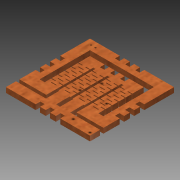
# Autodesk Inventor part: mech
Saved by Autodesk Inventor 2014 SP1 (Build 180222100, 222)
## iProperties
Created: 2015-02-17
Part Number: mech
Material: Wood (Cherry)
Document SubType Name: Modeling
Designer: Erin
Density: 0.63 g/cm^3
Appearance: Cherry - Natural Low Gloss
Author: Erin
Autodesk Inventor part; units mm, degrees
(part 1 of 2)
ref_plane "YZ Plane" through (0, 0, 0) normal (1, 0, 0) x (0, 1, 0)
ref_plane "XZ Plane" through (0, 0, 0) normal (0, 1, 0) x (-1, 0, 0)
ref_plane "XY Plane" through (0, 0, 0) normal (0, 0, 1) x (1, 0, 0)
sketch "slots" plane through (0, 0, 0) normal (0, 0, 1) x (1, 0, 0)
  line L0 (61.2067, 31.1821) -> (64.2567, 31.1821)
  line L1 (64.2567, 31.1821) -> (64.2567, 28.1071)
  line L2 (64.2567, 28.1071) -> (61.2067, 28.1071)
  line L3 (61.2067, 28.1071) -> (61.2067, 31.1821)
  line L4 (68.9317, 33.8834) -> (68.9317, 26.9198) construction
  line L5 (67.4067, 31.1821) -> (70.4567, 31.1821)
  line L6 (70.4567, 31.1821) -> (70.4567, 28.1071)
  line L7 (70.4567, 28.1071) -> (67.4067, 28.1071)
  line L8 (67.4067, 28.1071) -> (67.4067, 31.1821)
  line L9 (73.6067, 31.1821) -> (76.6567, 31.1821)
  line L10 (76.6567, 31.1821) -> (76.6567, 28.1071)
  line L11 (76.6567, 28.1071) -> (73.6067, 28.1071)
  line L12 (73.6067, 28.1071) -> (73.6067, 31.1821)
  line L13 (68.9317, 28.1071) -> (68.9317, 27.1937) construction
  point P0 (68.8645, 30.3856)
  dimension "d2" = 3.05
  dimension "d3" = 3.075
  dimension "d99" = 3.15
  dimension "d100" = 3.15
  measures "d2" distance of L1.end L2.end
  measures "d3" distance of L0.end L1.end
  measures "d99" distance between parallel lines of L8 L1
  measures "d100" distance between parallel lines of L12 L6
sketch "flexure" plane through (0, 0, 0) normal (0, 0, 1) x (1, 0, 0)
  line L0 (48.9032, 41.5133) -> (55.9032, 41.5133)
  line L1 (55.9032, 41.5133) -> (55.9032, 19.5133)
  line L2 (55.9032, 19.5133) -> (48.9032, 19.5133)
  line L3 (48.9032, 19.5133) -> (48.9032, 41.5133)
  line L4 (48.9032, 31.7633) -> (51.4486, 31.7633)
  line L5 (51.4486, 31.7633) -> (51.4486, 31.2633)
  line L6 (51.4486, 31.2633) -> (48.9032, 31.2633)
  line L7 (48.9032, 31.2633) -> (48.9032, 31.7633)
  line L8 (53.3577, 31.2633) -> (53.3577, 31.7633)
  line L9 (55.9032, 31.2633) -> (53.3577, 31.2633)
  line L10 (53.3577, 31.7633) -> (55.9032, 31.7633)
  line L11 (55.9032, 31.7633) -> (55.9032, 31.2633)
  line L12 (50.8123, 29.7633) -> (53.9941, 29.7633)
  line L13 (53.9941, 29.7633) -> (53.9941, 29.2633)
  line L14 (53.9941, 29.2633) -> (50.8123, 29.2633)
  line L15 (50.8123, 29.2633) -> (50.8123, 29.7633)
  line L16 (48.9032, 30.5133) -> (55.9032, 30.5133) construction
  line L17 (55.9032, 30.5133) -> (48.9032, 30.5133) construction
  line L18 (53.3577, 27.7633) -> (55.9032, 27.7633)
  line L19 (55.9032, 27.7633) -> (55.9032, 27.2633)
  line L20 (55.9032, 27.2633) -> (53.3577, 27.2633)
  line L21 (53.3577, 27.2633) -> (53.3577, 27.7633)
  line L22 (50.8123, 25.7633) -> (53.9941, 25.7633)
  line L23 (53.9941, 25.7633) -> (53.9941, 25.2633)
  line L24 (53.9941, 25.2633) -> (50.8123, 25.2633)
  line L25 (50.8123, 25.2633) -> (50.8123, 25.7633)
  line L26 (48.9032, 27.7633) -> (51.4486, 27.7633)
  line L27 (51.4486, 27.7633) -> (51.4486, 27.2633)
  line L28 (51.4486, 27.2633) -> (48.9032, 27.2633)
  line L29 (48.9032, 27.2633) -> (48.9032, 27.7633)
  line L30 (48.9032, 26.5133) -> (55.9032, 26.5133) construction
  line L31 (55.9032, 26.5133) -> (48.9032, 26.5133) construction
  line L32 (53.3577, 23.7633) -> (55.9032, 23.7633)
  line L33 (55.9032, 23.7633) -> (55.9032, 23.2633)
  line L34 (55.9032, 23.2633) -> (53.3577, 23.2633)
  line L35 (53.3577, 23.2633) -> (53.3577, 23.7633)
  line L36 (50.8123, 21.7633) -> (53.9941, 21.7633)
  line L37 (53.9941, 21.7633) -> (53.9941, 21.2633)
  line L38 (53.9941, 21.2633) -> (50.8123, 21.2633)
  line L39 (50.8123, 21.2633) -> (50.8123, 21.7633)
  line L40 (48.9032, 23.7633) -> (51.4486, 23.7633)
  line L41 (51.4486, 23.7633) -> (51.4486, 23.2633)
  line L42 (51.4486, 23.2633) -> (48.9032, 23.2633)
  line L43 (48.9032, 23.2633) -> (48.9032, 23.7633)
  line L44 (48.9032, 22.5133) -> (55.9032, 22.5133) construction
  line L45 (55.9032, 22.5133) -> (48.9032, 22.5133) construction
  line L46 (53.3577, 35.7633) -> (55.9032, 35.7633)
  line L47 (55.9032, 35.7633) -> (55.9032, 35.2633)
  line L48 (55.9032, 35.2633) -> (53.3577, 35.2633)
  line L49 (53.3577, 35.2633) -> (53.3577, 35.7633)
  line L50 (50.8123, 33.7633) -> (53.9941, 33.7633)
  line L51 (53.9941, 33.7633) -> (53.9941, 33.2633)
  line L52 (53.9941, 33.2633) -> (50.8123, 33.2633)
  line L53 (50.8123, 33.2633) -> (50.8123, 33.7633)
  line L54 (48.9032, 35.7633) -> (51.4486, 35.7633)
  line L55 (51.4486, 35.7633) -> (51.4486, 35.2633)
  line L56 (51.4486, 35.2633) -> (48.9032, 35.2633)
  line L57 (48.9032, 35.2633) -> (48.9032, 35.7633)
  line L58 (48.9032, 34.5133) -> (55.9032, 34.5133) construction
  line L59 (55.9032, 34.5133) -> (48.9032, 34.5133) construction
  line L60 (53.3577, 31.7633) -> (55.9032, 31.7633)
  line L61 (55.9032, 31.7633) -> (55.9032, 31.2633)
  line L62 (55.9032, 31.2633) -> (53.3577, 31.2633)
  line L63 (53.3577, 31.2633) -> (53.3577, 31.7633)
  line L64 (50.8123, 29.7633) -> (53.9941, 29.7633)
  line L65 (53.9941, 29.7633) -> (53.9941, 29.2633)
  line L66 (53.9941, 29.2633) -> (50.8123, 29.2633)
  line L67 (50.8123, 29.2633) -> (50.8123, 29.7633)
  line L68 (48.9032, 31.7633) -> (51.4486, 31.7633)
  line L69 (51.4486, 31.7633) -> (51.4486, 31.2633)
  line L70 (51.4486, 31.2633) -> (48.9032, 31.2633)
  line L71 (48.9032, 31.2633) -> (48.9032, 31.7633)
  line L72 (48.9032, 30.5133) -> (55.9032, 30.5133) construction
  line L73 (55.9032, 30.5133) -> (48.9032, 30.5133) construction
  line L74 (53.3577, 27.7633) -> (55.9032, 27.7633)
  line L75 (55.9032, 27.7633) -> (55.9032, 27.2633)
  line L76 (55.9032, 27.2633) -> (53.3577, 27.2633)
  line L77 (53.3577, 27.2633) -> (53.3577, 27.7633)
  line L78 (50.8123, 25.7633) -> (53.9941, 25.7633)
  line L79 (53.9941, 25.7633) -> (53.9941, 25.2633)
  line L80 (53.9941, 25.2633) -> (50.8123, 25.2633)
  line L81 (50.8123, 25.2633) -> (50.8123, 25.7633)
  line L82 (48.9032, 27.7633) -> (51.4486, 27.7633)
  line L83 (51.4486, 27.7633) -> (51.4486, 27.2633)
  line L84 (51.4486, 27.2633) -> (48.9032, 27.2633)
  line L85 (48.9032, 27.2633) -> (48.9032, 27.7633)
  line L86 (48.9032, 26.5133) -> (55.9032, 26.5133) construction
  line L87 (55.9032, 26.5133) -> (48.9032, 26.5133) construction
  line L88 (53.3577, 39.7633) -> (55.9032, 39.7633)
  line L89 (55.9032, 39.7633) -> (55.9032, 39.2633)
  line L90 (55.9032, 39.2633) -> (53.3577, 39.2633)
  line L91 (53.3577, 39.2633) -> (53.3577, 39.7633)
  line L92 (50.8123, 37.7633) -> (53.9941, 37.7633)
  line L93 (53.9941, 37.7633) -> (53.9941, 37.2633)
  line L94 (53.9941, 37.2633) -> (50.8123, 37.2633)
  line L95 (50.8123, 37.2633) -> (50.8123, 37.7633)
  line L96 (48.9032, 39.7633) -> (51.4486, 39.7633)
  line L97 (51.4486, 39.7633) -> (51.4486, 39.2633)
  line L98 (51.4486, 39.2633) -> (48.9032, 39.2633)
  line L99 (48.9032, 39.2633) -> (48.9032, 39.7633)
  line L100 (48.9032, 38.5133) -> (55.9032, 38.5133) construction
  line L101 (55.9032, 38.5133) -> (48.9032, 38.5133) construction
  line L102 (53.3577, 35.7633) -> (55.9032, 35.7633)
  line L103 (55.9032, 35.7633) -> (55.9032, 35.2633)
  line L104 (55.9032, 35.2633) -> (53.3577, 35.2633)
  line L105 (53.3577, 35.2633) -> (53.3577, 35.7633)
  line L106 (50.8123, 33.7633) -> (53.9941, 33.7633)
  line L107 (53.9941, 33.7633) -> (53.9941, 33.2633)
  line L108 (53.9941, 33.2633) -> (50.8123, 33.2633)
  line L109 (50.8123, 33.2633) -> (50.8123, 33.7633)
  line L110 (48.9032, 35.7633) -> (51.4486, 35.7633)
  line L111 (51.4486, 35.7633) -> (51.4486, 35.2633)
  line L112 (51.4486, 35.2633) -> (48.9032, 35.2633)
  line L113 (48.9032, 35.2633) -> (48.9032, 35.7633)
  line L114 (48.9032, 34.5133) -> (55.9032, 34.5133) construction
  line L115 (55.9032, 34.5133) -> (48.9032, 34.5133) construction
  line L116 (53.3577, 31.7633) -> (55.9032, 31.7633)
  line L117 (55.9032, 31.7633) -> (55.9032, 31.2633)
  line L118 (55.9032, 31.2633) -> (53.3577, 31.2633)
  line L119 (53.3577, 31.2633) -> (53.3577, 31.7633)
  line L120 (50.8123, 29.7633) -> (53.9941, 29.7633)
  line L121 (53.9941, 29.7633) -> (53.9941, 29.2633)
  line L122 (53.9941, 29.2633) -> (50.8123, 29.2633)
  line L123 (50.8123, 29.2633) -> (50.8123, 29.7633)
  line L124 (48.9032, 31.7633) -> (51.4486, 31.7633)
  line L125 (51.4486, 31.7633) -> (51.4486, 31.2633)
  line L126 (51.4486, 31.2633) -> (48.9032, 31.2633)
  line L127 (48.9032, 31.2633) -> (48.9032, 31.7633)
  line L128 (48.9032, 30.5133) -> (55.9032, 30.5133) construction
  line L129 (55.9032, 30.5133) -> (48.9032, 30.5133) construction
  line L130 (53.3577, 19.7633) -> (55.9032, 19.7633)
  line L131 (55.9032, 19.7633) -> (55.9032, 19.2633)
  line L132 (55.9032, 19.2633) -> (53.3577, 19.2633)
  line L133 (53.3577, 19.2633) -> (53.3577, 19.7633)
  line L134 (50.8123, 17.7633) -> (53.9941, 17.7633)
  line L135 (53.9941, 17.7633) -> (53.9941, 17.2633)
  line L136 (53.9941, 17.2633) -> (50.8123, 17.2633)
  line L137 (50.8123, 17.2633) -> (50.8123, 17.7633)
  line L138 (48.9032, 19.7633) -> (51.4486, 19.7633)
  line L139 (51.4486, 19.7633) -> (51.4486, 19.2633)
  line L140 (51.4486, 19.2633) -> (48.9032, 19.2633)
  line L141 (48.9032, 19.2633) -> (48.9032, 19.7633)
  line L142 (48.9032, 18.5133) -> (55.9032, 18.5133) construction
  line L143 (55.9032, 18.5133) -> (48.9032, 18.5133) construction
  line L144 (53.3577, 23.7633) -> (55.9032, 23.7633)
  line L145 (55.9032, 23.7633) -> (55.9032, 23.2633)
  line L146 (55.9032, 23.2633) -> (53.3577, 23.2633)
  line L147 (53.3577, 23.2633) -> (53.3577, 23.7633)
  line L148 (50.8123, 21.7633) -> (53.9941, 21.7633)
  line L149 (53.9941, 21.7633) -> (53.9941, 21.2633)
  line L150 (53.9941, 21.2633) -> (50.8123, 21.2633)
  line L151 (50.8123, 21.2633) -> (50.8123, 21.7633)
  line L152 (48.9032, 23.7633) -> (51.4486, 23.7633)
  line L153 (51.4486, 23.7633) -> (51.4486, 23.2633)
  line L154 (51.4486, 23.2633) -> (48.9032, 23.2633)
  line L155 (48.9032, 23.2633) -> (48.9032, 23.7633)
  line L156 (48.9032, 22.5133) -> (55.9032, 22.5133) construction
  line L157 (55.9032, 22.5133) -> (48.9032, 22.5133) construction
  line L158 (53.3577, 27.7633) -> (55.9032, 27.7633)
  line L159 (55.9032, 27.7633) -> (55.9032, 27.2633)
  line L160 (55.9032, 27.2633) -> (53.3577, 27.2633)
  line L161 (53.3577, 27.2633) -> (53.3577, 27.7633)
  line L162 (50.8123, 25.7633) -> (53.9941, 25.7633)
  line L163 (53.9941, 25.7633) -> (53.9941, 25.2633)
  line L164 (53.9941, 25.2633) -> (50.8123, 25.2633)
  line L165 (50.8123, 25.2633) -> (50.8123, 25.7633)
  line L166 (48.9032, 27.7633) -> (51.4486, 27.7633)
  line L167 (51.4486, 27.7633) -> (51.4486, 27.2633)
  line L168 (51.4486, 27.2633) -> (48.9032, 27.2633)
  line L169 (48.9032, 27.2633) -> (48.9032, 27.7633)
  line L170 (48.9032, 26.5133) -> (55.9032, 26.5133) construction
  line L171 (55.9032, 26.5133) -> (48.9032, 26.5133) construction
  line L172 (53.3577, 43.7633) -> (55.9032, 43.7633)
  line L173 (55.9032, 43.7633) -> (55.9032, 43.2633)
  line L174 (55.9032, 43.2633) -> (53.3577, 43.2633)
  line L175 (53.3577, 43.2633) -> (53.3577, 43.7633)
  line L176 (50.8123, 41.7633) -> (53.9941, 41.7633)
  line L177 (53.9941, 41.7633) -> (53.9941, 41.2633)
  line L178 (53.9941, 41.2633) -> (50.8123, 41.2633)
  line L179 (50.8123, 41.2633) -> (50.8123, 41.7633)
  line L180 (48.9032, 43.7633) -> (51.4486, 43.7633)
  line L181 (51.4486, 43.7633) -> (51.4486, 43.2633)
  line L182 (51.4486, 43.2633) -> (48.9032, 43.2633)
  line L183 (48.9032, 43.2633) -> (48.9032, 43.7633)
  line L184 (48.9032, 42.5133) -> (55.9032, 42.5133) construction
  line L185 (55.9032, 42.5133) -> (48.9032, 42.5133) construction
  line L186 (53.3577, 39.7633) -> (55.9032, 39.7633)
  line L187 (55.9032, 39.7633) -> (55.9032, 39.2633)
  line L188 (55.9032, 39.2633) -> (53.3577, 39.2633)
  line L189 (53.3577, 39.2633) -> (53.3577, 39.7633)
  line L190 (50.8123, 37.7633) -> (53.9941, 37.7633)
  line L191 (53.9941, 37.7633) -> (53.9941, 37.2633)
  line L192 (53.9941, 37.2633) -> (50.8123, 37.2633)
  line L193 (50.8123, 37.2633) -> (50.8123, 37.7633)
  line L194 (48.9032, 39.7633) -> (51.4486, 39.7633)
  line L195 (51.4486, 39.7633) -> (51.4486, 39.2633)
  line L196 (51.4486, 39.2633) -> (48.9032, 39.2633)
  line L197 (48.9032, 39.2633) -> (48.9032, 39.7633)
  line L198 (48.9032, 38.5133) -> (55.9032, 38.5133) construction
  line L199 (55.9032, 38.5133) -> (48.9032, 38.5133) construction
  line L200 (53.3577, 35.7633) -> (55.9032, 35.7633)
  line L201 (55.9032, 35.7633) -> (55.9032, 35.2633)
  line L202 (55.9032, 35.2633) -> (53.3577, 35.2633)
  line L203 (53.3577, 35.2633) -> (53.3577, 35.7633)
  line L204 (50.8123, 33.7633) -> (53.9941, 33.7633)
  line L205 (53.9941, 33.7633) -> (53.9941, 33.2633)
  line L206 (53.9941, 33.2633) -> (50.8123, 33.2633)
  line L207 (50.8123, 33.2633) -> (50.8123, 33.7633)
  line L208 (48.9032, 35.7633) -> (51.4486, 35.7633)
  line L209 (51.4486, 35.7633) -> (51.4486, 35.2633)
  line L210 (51.4486, 35.2633) -> (48.9032, 35.2633)
  line L211 (48.9032, 35.2633) -> (48.9032, 35.7633)
  line L212 (48.9032, 34.5133) -> (55.9032, 34.5133) construction
  line L213 (55.9032, 34.5133) -> (48.9032, 34.5133) construction
  line L214 (53.3577, 31.7633) -> (55.9032, 31.7633)
  line L215 (55.9032, 31.7633) -> (55.9032, 31.2633)
  line L216 (55.9032, 31.2633) -> (53.3577, 31.2633)
  line L217 (53.3577, 31.2633) -> (53.3577, 31.7633)
  line L218 (50.8123, 29.7633) -> (53.9941, 29.7633)
  line L219 (53.9941, 29.7633) -> (53.9941, 29.2633)
  line L220 (53.9941, 29.2633) -> (50.8123, 29.2633)
  line L221 (50.8123, 29.2633) -> (50.8123, 29.7633)
  line L222 (48.9032, 31.7633) -> (51.4486, 31.7633)
  line L223 (51.4486, 31.7633) -> (51.4486, 31.2633)
  line L224 (51.4486, 31.2633) -> (48.9032, 31.2633)
  line L225 (48.9032, 31.2633) -> (48.9032, 31.7633)
  line L226 (48.9032, 30.5133) -> (55.9032, 30.5133) construction
  line L227 (55.9032, 30.5133) -> (48.9032, 30.5133) construction
  point P0 (52.8239, 25.8216)
  dimension "d22" = 7
  dimension "d24" = 2.5455
  dimension "d27" = 4.4546
  dimension "d32" = 1.9091
  dimension "d33" = 3.1818
  dimension "d41" = 0.5
  dimension "d42" = 0.5
  dimension "d43" = 1.5
  dimension "d93" = 22
  dimension "d106" = 4
  dimension "d109" = 4
  dimension "d116" = 11.75
  measures "d22" distance of L1.end L2.end
  measures "d24" distance of L4.start L4.end
  measures "d27" distance of L6.end L9.end
  measures "d32" distance between parallel lines of L15 L3
  measures "d33" distance of L12.start L12.end
  measures "d41" distance of L4.end L5.end
  measures "d42" distance of L12.end L13.end
  measures "d43" distance between parallel lines of L12 L6
  measures "d93" distance of L0.end L1.end
  measures "d106" distance of L10.start L18.start
  measures "d109" distance of L10.start L46.start
  measures "d116" distance between parallel lines of L12 L0
sketch "Sketch1" plane through (0, 0, 0) normal (0, 0, 1) x (1, 0, 0)
  line L0 (-25, 25) -> (25, 25) construction
  line L1 (25, 25) -> (25, -25) construction
  line L2 (25, -25) -> (-25, -25) construction
  line L3 (-25, -25) -> (-25, 25) construction
  line L4 (-25, -25) -> (25, -25)
  line L5 (25, -25) -> (25, -19)
  line L6 (25, -19) -> (-25, -19)
  line L7 (-25, -19) -> (-25, -25)
  line L8 (0, 33.5916) -> (0, -39.9789) construction
  line L9 (-35.9054, 0) -> (42.6007, 0) construction
  line L10 (-25, 25) -> (25, 25)
  line L11 (25, 25) -> (25, 19)
  line L12 (25, 19) -> (-25, 19)
  line L13 (-25, 19) -> (-25, 25)
  line L14 (-25, 19) -> (-19, 19)
  line L15 (-19, 19) -> (-19, -17)
  line L16 (-19, -17) -> (-25, -17)
  line L17 (-25, -17) -> (-25, 19)
  line L18 (-19, -17) -> (-9, -17)
  line L19 (-9, -17) -> (-9, -11)
  line L20 (-9, -11) -> (-19, -11)
  line L21 (-19, -11) -> (-19, -17)
  line L22 (25, 19) -> (19, 19)
  line L23 (19, 19) -> (19, -17)
  line L24 (19, -17) -> (25, -17)
  line L25 (25, -17) -> (25, 19)
  line L26 (19, -17) -> (9, -17)
  line L27 (9, -17) -> (9, -11)
  line L28 (9, -11) -> (19, -11)
  line L29 (19, -11) -> (19, -17)
  line L30 (-16, 16) -> (16, 16)
  line L31 (16, 16) -> (16, 11)
  line L32 (16, 11) -> (-16, 11)
  line L33 (-16, 11) -> (-16, 16)
  line L34 (-7.2, -11) -> (-1.2, -11)
  line L35 (-1.2, -11) -> (-1.2, -19)
  line L36 (-1.2, -19) -> (-7.2, -19)
  line L37 (-7.2, -19) -> (-7.2, -11)
  line L38 (1.2, -11) -> (7.2, -11)
  line L39 (7.2, -11) -> (7.2, -19)
  line L40 (7.2, -19) -> (1.2, -19)
  line L41 (1.2, -19) -> (1.2, -11)
  line L42 (-68.1542, 16.5688) -> (-29.44, 16.5688) construction
  line L43 (-29.44, 16.5688) -> (-29.44, -5.0786) construction
  line L44 (-29.44, -5.0786) -> (-68.1542, -5.0786) construction
  line L45 (-68.1542, -5.0786) -> (-68.1542, 16.5688) construction
  circle A0 centre (-21.2866, 22) radius 0.5
  circle A1 centre (-18.6754, 22) radius 0.5
  line L46 (-7.725, 25) -> (-4.675, 25)
  line L47 (-4.675, 25) -> (-4.675, 21.925)
  line L48 (-4.675, 21.925) -> (-7.725, 21.925)
  line L49 (-7.725, 21.925) -> (-7.725, 25)
  line L50 (0, 27.7013) -> (0, 20.7377) construction
  line L51 (-1.525, 25) -> (1.525, 25)
  line L52 (1.525, 25) -> (1.525, 21.925)
  line L53 (1.525, 21.925) -> (-1.525, 21.925)
  line L54 (-1.525, 21.925) -> (-1.525, 25)
  line L55 (4.675, 25) -> (7.725, 25)
  line L56 (7.725, 25) -> (7.725, 21.925)
  line L57 (7.725, 21.925) -> (4.675, 21.925)
  line L58 (4.675, 21.925) -> (4.675, 25)
  line L59 (0, 21.925) -> (0, 21.0116) construction
  line L60 (-7.725, -21.925) -> (-4.675, -21.925)
  line L61 (-4.675, -21.925) -> (-4.675, -25)
  line L62 (-4.675, -25) -> (-7.725, -25)
  line L63 (-7.725, -25) -> (-7.725, -21.925)
  line L64 (0, -19.2237) -> (0, -26.1873) construction
  line L65 (-1.525, -21.925) -> (1.525, -21.925)
  line L66 (1.525, -21.925) -> (1.525, -25)
  line L67 (1.525, -25) -> (-1.525, -25)
  line L68 (-1.525, -25) -> (-1.525, -21.925)
  line L69 (4.675, -21.925) -> (7.725, -21.925)
  line L70 (7.725, -21.925) -> (7.725, -25)
  line L71 (7.725, -25) -> (4.675, -25)
  line L72 (4.675, -25) -> (4.675, -21.925)
  line L73 (0, -25) -> (0, -25.9134) construction
  line L74 (-25, -7.725) -> (-25, -4.675)
  line L75 (-25, -4.675) -> (-21.925, -4.675)
  line L76 (-21.925, -4.675) -> (-21.925, -7.725)
  line L77 (-21.925, -7.725) -> (-25, -7.725)
  line L78 (-27.7013, 0) -> (-20.7377, 0) construction
  line L79 (-25, -1.525) -> (-25, 1.525)
  line L80 (-25, 1.525) -> (-21.925, 1.525)
  line L81 (-21.925, 1.525) -> (-21.925, -1.525)
  line L82 (-21.925, -1.525) -> (-25, -1.525)
  line L83 (-25, 4.675) -> (-25, 7.725)
  line L84 (-25, 7.725) -> (-21.925, 7.725)
  line L85 (-21.925, 7.725) -> (-21.925, 4.675)
  line L86 (-21.925, 4.675) -> (-25, 4.675)
  line L87 (-21.925, 0) -> (-21.0116, 0) construction
  line L88 (21.925, -7.725) -> (21.925, -4.675)
  line L89 (21.925, -4.675) -> (25, -4.675)
  line L90 (25, -4.675) -> (25, -7.725)
  line L91 (25, -7.725) -> (21.925, -7.725)
  line L92 (19.2237, 0) -> (26.1873, 0) construction
  line L93 (21.925, -1.525) -> (21.925, 1.525)
  line L94 (21.925, 1.525) -> (25, 1.525)
  line L95 (25, 1.525) -> (25, -1.525)
  line L96 (25, -1.525) -> (21.925, -1.525)
  line L97 (21.925, 4.675) -> (21.925, 7.725)
  line L98 (21.925, 7.725) -> (25, 7.725)
  line L99 (25, 7.725) -> (25, 4.675)
  line L100 (25, 4.675) -> (21.925, 4.675)
  line L101 (25, 0) -> (25.9134, 0) construction
  line L102 (-16, 11) -> (-9, 11)
  line L103 (-9, 11) -> (-9, -11)
  line L104 (-9, -11) -> (-16, -11)
  line L105 (-16, -11) -> (-16, 11)
  line L106 (-16, 1.25) -> (-13.4545, 1.25)
  line L107 (-13.4545, 1.25) -> (-13.4545, 0.75)
  line L108 (-13.4545, 0.75) -> (-16, 0.75)
  line L109 (-16, 0.75) -> (-16, 1.25)
  line L110 (-11.5455, 0.75) -> (-11.5455, 1.25)
  line L111 (-9, 0.75) -> (-11.5455, 0.75)
  line L112 (-11.5455, 1.25) -> (-9, 1.25)
  line L113 (-9, 1.25) -> (-9, 0.75)
  line L114 (-14.0909, -0.75) -> (-10.9091, -0.75)
  line L115 (-10.9091, -0.75) -> (-10.9091, -1.25)
  line L116 (-10.9091, -1.25) -> (-14.0909, -1.25)
  line L117 (-14.0909, -1.25) -> (-14.0909, -0.75)
  line L118 (-16, 0) -> (-9, 0) construction
  line L119 (-9, 0) -> (-16, 0) construction
  line L120 (-11.5455, -2.75) -> (-9, -2.75)
  line L121 (-9, -2.75) -> (-9, -3.25)
  line L122 (-9, -3.25) -> (-11.5455, -3.25)
  line L123 (-11.5455, -3.25) -> (-11.5455, -2.75)
  line L124 (-14.0909, -4.75) -> (-10.9091, -4.75)
  line L125 (-10.9091, -4.75) -> (-10.9091, -5.25)
  line L126 (-10.9091, -5.25) -> (-14.0909, -5.25)
  line L127 (-14.0909, -5.25) -> (-14.0909, -4.75)
  line L128 (-16, -2.75) -> (-13.4545, -2.75)
  line L129 (-13.4545, -2.75) -> (-13.4545, -3.25)
  line L130 (-13.4545, -3.25) -> (-16, -3.25)
  line L131 (-16, -3.25) -> (-16, -2.75)
  line L132 (-16, -4) -> (-9, -4) construction
  line L133 (-9, -4) -> (-16, -4) construction
  line L134 (-11.5455, -6.75) -> (-9, -6.75)
  line L135 (-9, -6.75) -> (-9, -7.25)
  line L136 (-9, -7.25) -> (-11.5455, -7.25)
  line L137 (-11.5455, -7.25) -> (-11.5455, -6.75)
  line L138 (-14.0909, -8.75) -> (-10.9091, -8.75)
  line L139 (-10.9091, -8.75) -> (-10.9091, -9.25)
  line L140 (-10.9091, -9.25) -> (-14.0909, -9.25)
  line L141 (-14.0909, -9.25) -> (-14.0909, -8.75)
  line L142 (-16, -6.75) -> (-13.4545, -6.75)
  line L143 (-13.4545, -6.75) -> (-13.4545, -7.25)
  line L144 (-13.4545, -7.25) -> (-16, -7.25)
  line L145 (-16, -7.25) -> (-16, -6.75)
  line L146 (-16, -8) -> (-9, -8) construction
  line L147 (-9, -8) -> (-16, -8) construction
  line L148 (-11.5455, 5.25) -> (-9, 5.25)
  line L149 (-9, 5.25) -> (-9, 4.75)
  line L150 (-9, 4.75) -> (-11.5455, 4.75)
  line L151 (-11.5455, 4.75) -> (-11.5455, 5.25)
  line L152 (-14.0909, 3.25) -> (-10.9091, 3.25)
  line L153 (-10.9091, 3.25) -> (-10.9091, 2.75)
  line L154 (-10.9091, 2.75) -> (-14.0909, 2.75)
  line L155 (-14.0909, 2.75) -> (-14.0909, 3.25)
  line L156 (-16, 5.25) -> (-13.4545, 5.25)
  line L157 (-13.4545, 5.25) -> (-13.4545, 4.75)
  line L158 (-13.4545, 4.75) -> (-16, 4.75)
  line L159 (-16, 4.75) -> (-16, 5.25)
  line L160 (-16, 4) -> (-9, 4) construction
  line L161 (-9, 4) -> (-16, 4) construction
  line L162 (-11.5455, 1.25) -> (-9, 1.25)
  line L163 (-9, 1.25) -> (-9, 0.75)
  line L164 (-9, 0.75) -> (-11.5455, 0.75)
  line L165 (-11.5455, 0.75) -> (-11.5455, 1.25)
  line L166 (-14.0909, -0.75) -> (-10.9091, -0.75)
  line L167 (-10.9091, -0.75) -> (-10.9091, -1.25)
  line L168 (-10.9091, -1.25) -> (-14.0909, -1.25)
  line L169 (-14.0909, -1.25) -> (-14.0909, -0.75)
  line L170 (-16, 1.25) -> (-13.4545, 1.25)
  line L171 (-13.4545, 1.25) -> (-13.4545, 0.75)
  line L172 (-13.4545, 0.75) -> (-16, 0.75)
  line L173 (-16, 0.75) -> (-16, 1.25)
  line L174 (-16, 0) -> (-9, 0) construction
  line L175 (-9, 0) -> (-16, 0) construction
  line L176 (-11.5455, -2.75) -> (-9, -2.75)
  line L177 (-9, -2.75) -> (-9, -3.25)
  line L178 (-9, -3.25) -> (-11.5455, -3.25)
  line L179 (-11.5455, -3.25) -> (-11.5455, -2.75)
  line L180 (-14.0909, -4.75) -> (-10.9091, -4.75)
  line L181 (-10.9091, -4.75) -> (-10.9091, -5.25)
  line L182 (-10.9091, -5.25) -> (-14.0909, -5.25)
  line L183 (-14.0909, -5.25) -> (-14.0909, -4.75)
  line L184 (-16, -2.75) -> (-13.4545, -2.75)
  line L185 (-13.4545, -2.75) -> (-13.4545, -3.25)
  line L186 (-13.4545, -3.25) -> (-16, -3.25)
  line L187 (-16, -3.25) -> (-16, -2.75)
  line L188 (-16, -4) -> (-9, -4) construction
  line L189 (-9, -4) -> (-16, -4) construction
  line L190 (-11.5455, 9.25) -> (-9, 9.25)
  line L191 (-9, 9.25) -> (-9, 8.75)
  line L192 (-9, 8.75) -> (-11.5455, 8.75)
  line L193 (-11.5455, 8.75) -> (-11.5455, 9.25)
  line L194 (-14.0909, 7.25) -> (-10.9091, 7.25)
  line L195 (-10.9091, 7.25) -> (-10.9091, 6.75)
  line L196 (-10.9091, 6.75) -> (-14.0909, 6.75)
  line L197 (-14.0909, 6.75) -> (-14.0909, 7.25)
  line L198 (-16, 9.25) -> (-13.4545, 9.25)
  line L199 (-13.4545, 9.25) -> (-13.4545, 8.75)
  line L200 (-13.4545, 8.75) -> (-16, 8.75)
  line L201 (-16, 8.75) -> (-16, 9.25)
  line L202 (-16, 8) -> (-9, 8) construction
  line L203 (-9, 8) -> (-16, 8) construction
  line L204 (-11.5455, 5.25) -> (-9, 5.25)
  line L205 (-9, 5.25) -> (-9, 4.75)
  line L206 (-9, 4.75) -> (-11.5455, 4.75)
  line L207 (-11.5455, 4.75) -> (-11.5455, 5.25)
  line L208 (-14.0909, 3.25) -> (-10.9091, 3.25)
  line L209 (-10.9091, 3.25) -> (-10.9091, 2.75)
  line L210 (-10.9091, 2.75) -> (-14.0909, 2.75)
  line L211 (-14.0909, 2.75) -> (-14.0909, 3.25)
  line L212 (-16, 5.25) -> (-13.4545, 5.25)
  line L213 (-13.4545, 5.25) -> (-13.4545, 4.75)
  line L214 (-13.4545, 4.75) -> (-16, 4.75)
  line L215 (-16, 4.75) -> (-16, 5.25)
  line L216 (-16, 4) -> (-9, 4) construction
  line L217 (-9, 4) -> (-16, 4) construction
  line L218 (-11.5455, 1.25) -> (-9, 1.25)
  line L219 (-9, 1.25) -> (-9, 0.75)
  line L220 (-9, 0.75) -> (-11.5455, 0.75)
  line L221 (-11.5455, 0.75) -> (-11.5455, 1.25)
  line L222 (-14.0909, -0.75) -> (-10.9091, -0.75)
  line L223 (-10.9091, -0.75) -> (-10.9091, -1.25)
  line L224 (-10.9091, -1.25) -> (-14.0909, -1.25)
  line L225 (-14.0909, -1.25) -> (-14.0909, -0.75)
  line L226 (-16, 1.25) -> (-13.4545, 1.25)
  line L227 (-13.4545, 1.25) -> (-13.4545, 0.75)
  line L228 (-13.4545, 0.75) -> (-16, 0.75)
  line L229 (-16, 0.75) -> (-16, 1.25)
  line L230 (-16, 0) -> (-9, 0) construction
  line L231 (-9, 0) -> (-16, 0) construction
  line L232 (-11.5455, -10.75) -> (-9, -10.75)
  line L233 (-9, -10.75) -> (-9, -11.25)
  line L234 (-9, -11.25) -> (-11.5455, -11.25)
  line L235 (-11.5455, -11.25) -> (-11.5455, -10.75)
  line L236 (-14.0909, -12.75) -> (-10.9091, -12.75)
  line L237 (-10.9091, -12.75) -> (-10.9091, -13.25)
  line L238 (-10.9091, -13.25) -> (-14.0909, -13.25)
  line L239 (-14.0909, -13.25) -> (-14.0909, -12.75)
  line L240 (-16, -10.75) -> (-13.4545, -10.75)
  line L241 (-13.4545, -10.75) -> (-13.4545, -11.25)
  line L242 (-13.4545, -11.25) -> (-16, -11.25)
  line L243 (-16, -11.25) -> (-16, -10.75)
  line L244 (-16, -12) -> (-9, -12) construction
  line L245 (-9, -12) -> (-16, -12) construction
  line L246 (-11.5455, -6.75) -> (-9, -6.75)
  line L247 (-9, -6.75) -> (-9, -7.25)
  line L248 (-9, -7.25) -> (-11.5455, -7.25)
  line L249 (-11.5455, -7.25) -> (-11.5455, -6.75)
  line L250 (-14.0909, -8.75) -> (-10.9091, -8.75)
  line L251 (-10.9091, -8.75) -> (-10.9091, -9.25)
  line L252 (-10.9091, -9.25) -> (-14.0909, -9.25)
  line L253 (-14.0909, -9.25) -> (-14.0909, -8.75)
  line L254 (-16, -6.75) -> (-13.4545, -6.75)
  line L255 (-13.4545, -6.75) -> (-13.4545, -7.25)
  line L256 (-13.4545, -7.25) -> (-16, -7.25)
  line L257 (-16, -7.25) -> (-16, -6.75)
  line L258 (-16, -8) -> (-9, -8) construction
  line L259 (-9, -8) -> (-16, -8) construction
  line L260 (-11.5455, -2.75) -> (-9, -2.75)
  line L261 (-9, -2.75) -> (-9, -3.25)
  line L262 (-9, -3.25) -> (-11.5455, -3.25)
  line L263 (-11.5455, -3.25) -> (-11.5455, -2.75)
  line L264 (-14.0909, -4.75) -> (-10.9091, -4.75)
  line L265 (-10.9091, -4.75) -> (-10.9091, -5.25)
  line L266 (-10.9091, -5.25) -> (-14.0909, -5.25)
  line L267 (-14.0909, -5.25) -> (-14.0909, -4.75)
  line L268 (-16, -2.75) -> (-13.4545, -2.75)
  line L269 (-13.4545, -2.75) -> (-13.4545, -3.25)
  line L270 (-13.4545, -3.25) -> (-16, -3.25)
  line L271 (-16, -3.25) -> (-16, -2.75)
  line L272 (-16, -4) -> (-9, -4) construction
  line L273 (-9, -4) -> (-16, -4) construction
  line L274 (-11.5455, 13.25) -> (-9, 13.25)
  line L275 (-9, 13.25) -> (-9, 12.75)
  line L276 (-9, 12.75) -> (-11.5455, 12.75)
  line L277 (-11.5455, 12.75) -> (-11.5455, 13.25)
  line L278 (-14.0909, 11.25) -> (-10.9091, 11.25)
  line L279 (-10.9091, 11.25) -> (-10.9091, 10.75)
  line L280 (-10.9091, 10.75) -> (-14.0909, 10.75)
  line L281 (-14.0909, 10.75) -> (-14.0909, 11.25)
  line L282 (-16, 13.25) -> (-13.4545, 13.25)
  line L283 (-13.4545, 13.25) -> (-13.4545, 12.75)
  line L284 (-13.4545, 12.75) -> (-16, 12.75)
  line L285 (-16, 12.75) -> (-16, 13.25)
  line L286 (-16, 12) -> (-9, 12) construction
  line L287 (-9, 12) -> (-16, 12) construction
  line L288 (-11.5455, 9.25) -> (-9, 9.25)
  line L289 (-9, 9.25) -> (-9, 8.75)
  line L290 (-9, 8.75) -> (-11.5455, 8.75)
  line L291 (-11.5455, 8.75) -> (-11.5455, 9.25)
  line L292 (-14.0909, 7.25) -> (-10.9091, 7.25)
  line L293 (-10.9091, 7.25) -> (-10.9091, 6.75)
  line L294 (-10.9091, 6.75) -> (-14.0909, 6.75)
  line L295 (-14.0909, 6.75) -> (-14.0909, 7.25)
  line L296 (-16, 9.25) -> (-13.4545, 9.25)
  line L297 (-13.4545, 9.25) -> (-13.4545, 8.75)
  line L298 (-13.4545, 8.75) -> (-16, 8.75)
  line L299 (-16, 8.75) -> (-16, 9.25)
  line L300 (-16, 8) -> (-9, 8) construction
  line L301 (-9, 8) -> (-16, 8) construction
  line L302 (-11.5455, 5.25) -> (-9, 5.25)
  line L303 (-9, 5.25) -> (-9, 4.75)
  line L304 (-9, 4.75) -> (-11.5455, 4.75)
  line L305 (-11.5455, 4.75) -> (-11.5455, 5.25)
  line L306 (-14.0909, 3.25) -> (-10.9091, 3.25)
  line L307 (-10.9091, 3.25) -> (-10.9091, 2.75)
  line L308 (-10.9091, 2.75) -> (-14.0909, 2.75)
  line L309 (-14.0909, 2.75) -> (-14.0909, 3.25)
  line L310 (-16, 5.25) -> (-13.4545, 5.25)
  line L311 (-13.4545, 5.25) -> (-13.4545, 4.75)
  line L312 (-13.4545, 4.75) -> (-16, 4.75)
  line L313 (-16, 4.75) -> (-16, 5.25)
  line L314 (-16, 4) -> (-9, 4) construction
  line L315 (-9, 4) -> (-16, 4) construction
  line L316 (-11.5455, 1.25) -> (-9, 1.25)
  line L317 (-9, 1.25) -> (-9, 0.75)
  line L318 (-9, 0.75) -> (-11.5455, 0.75)
  line L319 (-11.5455, 0.75) -> (-11.5455, 1.25)
  line L320 (-14.0909, -0.75) -> (-10.9091, -0.75)
  line L321 (-10.9091, -0.75) -> (-10.9091, -1.25)
  line L322 (-10.9091, -1.25) -> (-14.0909, -1.25)
  line L323 (-14.0909, -1.25) -> (-14.0909, -0.75)
  line L324 (-16, 1.25) -> (-13.4545, 1.25)
  line L325 (-13.4545, 1.25) -> (-13.4545, 0.75)
  line L326 (-13.4545, 0.75) -> (-16, 0.75)
  line L327 (-16, 0.75) -> (-16, 1.25)
  line L328 (-16, 0) -> (-9, 0) construction
  line L329 (-9, 0) -> (-16, 0) construction
  line L330 (9, 11) -> (16, 11)
  line L331 (16, 11) -> (16, -11)
  line L332 (16, -11) -> (9, -11)
  line L333 (9, -11) -> (9, 11)
  line L334 (9, 1.25) -> (11.5455, 1.25)
  line L335 (11.5455, 1.25) -> (11.5455, 0.75)
  line L336 (11.5455, 0.75) -> (9, 0.75)
  line L337 (9, 0.75) -> (9, 1.25)
  line L338 (13.4545, 0.75) -> (13.4545, 1.25)
  line L339 (16, 0.75) -> (13.4545, 0.75)
  line L340 (13.4545, 1.25) -> (16, 1.25)
  line L341 (16, 1.25) -> (16, 0.75)
  line L342 (10.9091, -0.75) -> (14.0909, -0.75)
  line L343 (14.0909, -0.75) -> (14.0909, -1.25)
  line L344 (14.0909, -1.25) -> (10.9091, -1.25)
  line L345 (10.9091, -1.25) -> (10.9091, -0.75)
  line L346 (9, 0) -> (16, 0) construction
  line L347 (16, 0) -> (9, 0) construction
  line L348 (13.4545, -2.75) -> (16, -2.75)
  line L349 (16, -2.75) -> (16, -3.25)
  line L350 (16, -3.25) -> (13.4545, -3.25)
  line L351 (13.4545, -3.25) -> (13.4545, -2.75)
  line L352 (10.9091, -4.75) -> (14.0909, -4.75)
  line L353 (14.0909, -4.75) -> (14.0909, -5.25)
  line L354 (14.0909, -5.25) -> (10.9091, -5.25)
  line L355 (10.9091, -5.25) -> (10.9091, -4.75)
  line L356 (9, -2.75) -> (11.5455, -2.75)
  line L357 (11.5455, -2.75) -> (11.5455, -3.25)
  line L358 (11.5455, -3.25) -> (9, -3.25)
  line L359 (9, -3.25) -> (9, -2.75)
  line L360 (9, -4) -> (16, -4) construction
  line L361 (16, -4) -> (9, -4) construction
  line L362 (13.4545, -6.75) -> (16, -6.75)
  line L363 (16, -6.75) -> (16, -7.25)
  line L364 (16, -7.25) -> (13.4545, -7.25)
  line L365 (13.4545, -7.25) -> (13.4545, -6.75)
  line L366 (10.9091, -8.75) -> (14.0909, -8.75)
  line L367 (14.0909, -8.75) -> (14.0909, -9.25)
  line L368 (14.0909, -9.25) -> (10.9091, -9.25)
  line L369 (10.9091, -9.25) -> (10.9091, -8.75)
  line L370 (9, -6.75) -> (11.5455, -6.75)
  line L371 (11.5455, -6.75) -> (11.5455, -7.25)
  line L372 (11.5455, -7.25) -> (9, -7.25)
  line L373 (9, -7.25) -> (9, -6.75)
  line L374 (9, -8) -> (16, -8) construction
  line L375 (16, -8) -> (9, -8) construction
  line L376 (13.4545, 5.25) -> (16, 5.25)
  line L377 (16, 5.25) -> (16, 4.75)
  line L378 (16, 4.75) -> (13.4545, 4.75)
  line L379 (13.4545, 4.75) -> (13.4545, 5.25)
  line L380 (10.9091, 3.25) -> (14.0909, 3.25)
  line L381 (14.0909, 3.25) -> (14.0909, 2.75)
  line L382 (14.0909, 2.75) -> (10.9091, 2.75)
  line L383 (10.9091, 2.75) -> (10.9091, 3.25)
  line L384 (9, 5.25) -> (11.5455, 5.25)
  line L385 (11.5455, 5.25) -> (11.5455, 4.75)
  line L386 (11.5455, 4.75) -> (9, 4.75)
  line L387 (9, 4.75) -> (9, 5.25)
  line L388 (9, 4) -> (16, 4) construction
  line L389 (16, 4) -> (9, 4) construction
  line L390 (13.4545, 1.25) -> (16, 1.25)
  line L391 (16, 1.25) -> (16, 0.75)
  line L392 (16, 0.75) -> (13.4545, 0.75)
  line L393 (13.4545, 0.75) -> (13.4545, 1.25)
  line L394 (10.9091, -0.75) -> (14.0909, -0.75)
  line L395 (14.0909, -0.75) -> (14.0909, -1.25)
  line L396 (14.0909, -1.25) -> (10.9091, -1.25)
  line L397 (10.9091, -1.25) -> (10.9091, -0.75)
  line L398 (9, 1.25) -> (11.5455, 1.25)
  line L399 (11.5455, 1.25) -> (11.5455, 0.75)
  line L400 (11.5455, 0.75) -> (9, 0.75)
  line L401 (9, 0.75) -> (9, 1.25)
  line L402 (9, 0) -> (16, 0) construction
  line L403 (16, 0) -> (9, 0) construction
  line L404 (13.4545, -2.75) -> (16, -2.75)
  line L405 (16, -2.75) -> (16, -3.25)
  line L406 (16, -3.25) -> (13.4545, -3.25)
  line L407 (13.4545, -3.25) -> (13.4545, -2.75)
  line L408 (10.9091, -4.75) -> (14.0909, -4.75)
  line L409 (14.0909, -4.75) -> (14.0909, -5.25)
  line L410 (14.0909, -5.25) -> (10.9091, -5.25)
  line L411 (10.9091, -5.25) -> (10.9091, -4.75)
  line L412 (9, -2.75) -> (11.5455, -2.75)
  line L413 (11.5455, -2.75) -> (11.5455, -3.25)
  line L414 (11.5455, -3.25) -> (9, -3.25)
  line L415 (9, -3.25) -> (9, -2.75)
  line L416 (9, -4) -> (16, -4) construction
  line L417 (16, -4) -> (9, -4) construction
  line L418 (13.4545, 9.25) -> (16, 9.25)
  line L419 (16, 9.25) -> (16, 8.75)
  line L420 (16, 8.75) -> (13.4545, 8.75)
  line L421 (13.4545, 8.75) -> (13.4545, 9.25)
  line L422 (10.9091, 7.25) -> (14.0909, 7.25)
  line L423 (14.0909, 7.25) -> (14.0909, 6.75)
  line L424 (14.0909, 6.75) -> (10.9091, 6.75)
  line L425 (10.9091, 6.75) -> (10.9091, 7.25)
  line L426 (9, 9.25) -> (11.5455, 9.25)
  line L427 (11.5455, 9.25) -> (11.5455, 8.75)
  line L428 (11.5455, 8.75) -> (9, 8.75)
  line L429 (9, 8.75) -> (9, 9.25)
  line L430 (9, 8) -> (16, 8) construction
  line L431 (16, 8) -> (9, 8) construction
  line L432 (13.4545, 5.25) -> (16, 5.25)
  line L433 (16, 5.25) -> (16, 4.75)
  line L434 (16, 4.75) -> (13.4545, 4.75)
  line L435 (13.4545, 4.75) -> (13.4545, 5.25)
  line L436 (10.9091, 3.25) -> (14.0909, 3.25)
  line L437 (14.0909, 3.25) -> (14.0909, 2.75)
  line L438 (14.0909, 2.75) -> (10.9091, 2.75)
  line L439 (10.9091, 2.75) -> (10.9091, 3.25)
  line L440 (9, 5.25) -> (11.5455, 5.25)
  line L441 (11.5455, 5.25) -> (11.5455, 4.75)
  line L442 (11.5455, 4.75) -> (9, 4.75)
  line L443 (9, 4.75) -> (9, 5.25)
  line L444 (9, 4) -> (16, 4) construction
  line L445 (16, 4) -> (9, 4) construction
  line L446 (13.4545, 1.25) -> (16, 1.25)
  line L447 (16, 1.25) -> (16, 0.75)
  line L448 (16, 0.75) -> (13.4545, 0.75)
  line L449 (13.4545, 0.75) -> (13.4545, 1.25)
  line L450 (10.9091, -0.75) -> (14.0909, -0.75)
  line L451 (14.0909, -0.75) -> (14.0909, -1.25)
  line L452 (14.0909, -1.25) -> (10.9091, -1.25)
  line L453 (10.9091, -1.25) -> (10.9091, -0.75)
  line L454 (9, 1.25) -> (11.5455, 1.25)
  line L455 (11.5455, 1.25) -> (11.5455, 0.75)
  line L456 (11.5455, 0.75) -> (9, 0.75)
  line L457 (9, 0.75) -> (9, 1.25)
  line L458 (9, 0) -> (16, 0) construction
  line L459 (16, 0) -> (9, 0) construction
  line L460 (13.4545, -10.75) -> (16, -10.75)
  line L461 (16, -10.75) -> (16, -11.25)
  line L462 (16, -11.25) -> (13.4545, -11.25)
  line L463 (13.4545, -11.25) -> (13.4545, -10.75)
  line L464 (10.9091, -12.75) -> (14.0909, -12.75)
  line L465 (14.0909, -12.75) -> (14.0909, -13.25)
  line L466 (14.0909, -13.25) -> (10.9091, -13.25)
  line L467 (10.9091, -13.25) -> (10.9091, -12.75)
  line L468 (9, -10.75) -> (11.5455, -10.75)
  line L469 (11.5455, -10.75) -> (11.5455, -11.25)
  line L470 (11.5455, -11.25) -> (9, -11.25)
  line L471 (9, -11.25) -> (9, -10.75)
  line L472 (9, -12) -> (16, -12) construction
  line L473 (16, -12) -> (9, -12) construction
  line L474 (13.4545, -6.75) -> (16, -6.75)
  line L475 (16, -6.75) -> (16, -7.25)
  line L476 (16, -7.25) -> (13.4545, -7.25)
  line L477 (13.4545, -7.25) -> (13.4545, -6.75)
  line L478 (10.9091, -8.75) -> (14.0909, -8.75)
  line L479 (14.0909, -8.75) -> (14.0909, -9.25)
  line L480 (14.0909, -9.25) -> (10.9091, -9.25)
  line L481 (10.9091, -9.25) -> (10.9091, -8.75)
  line L482 (9, -6.75) -> (11.5455, -6.75)
  line L483 (11.5455, -6.75) -> (11.5455, -7.25)
  line L484 (11.5455, -7.25) -> (9, -7.25)
  line L485 (9, -7.25) -> (9, -6.75)
  line L486 (9, -8) -> (16, -8) construction
  line L487 (16, -8) -> (9, -8) construction
  line L488 (13.4545, -2.75) -> (16, -2.75)
  line L489 (16, -2.75) -> (16, -3.25)
  line L490 (16, -3.25) -> (13.4545, -3.25)
  line L491 (13.4545, -3.25) -> (13.4545, -2.75)
  line L492 (10.9091, -4.75) -> (14.0909, -4.75)
  line L493 (14.0909, -4.75) -> (14.0909, -5.25)
  line L494 (14.0909, -5.25) -> (10.9091, -5.25)
  line L495 (10.9091, -5.25) -> (10.9091, -4.75)
  line L496 (9, -2.75) -> (11.5455, -2.75)
  line L497 (11.5455, -2.75) -> (11.5455, -3.25)
  line L498 (11.5455, -3.25) -> (9, -3.25)
  line L499 (9, -3.25) -> (9, -2.75)
  line L500 (9, -4) -> (16, -4) construction
  line L501 (16, -4) -> (9, -4) construction
  line L502 (13.4545, 13.25) -> (16, 13.25)
  line L503 (16, 13.25) -> (16, 12.75)
  line L504 (16, 12.75) -> (13.4545, 12.75)
  line L505 (13.4545, 12.75) -> (13.4545, 13.25)
  line L506 (10.9091, 11.25) -> (14.0909, 11.25)
  line L507 (14.0909, 11.25) -> (14.0909, 10.75)
  line L508 (14.0909, 10.75) -> (10.9091, 10.75)
  line L509 (10.9091, 10.75) -> (10.9091, 11.25)
  line L510 (9, 13.25) -> (11.5455, 13.25)
  line L511 (11.5455, 13.25) -> (11.5455, 12.75)
  line L512 (11.5455, 12.75) -> (9, 12.75)
  line L513 (9, 12.75) -> (9, 13.25)
  line L514 (9, 12) -> (16, 12) construction
  line L515 (16, 12) -> (9, 12) construction
  line L516 (13.4545, 9.25) -> (16, 9.25)
  line L517 (16, 9.25) -> (16, 8.75)
  line L518 (16, 8.75) -> (13.4545, 8.75)
  line L519 (13.4545, 8.75) -> (13.4545, 9.25)
  line L520 (10.9091, 7.25) -> (14.0909, 7.25)
  line L521 (14.0909, 7.25) -> (14.0909, 6.75)
  line L522 (14.0909, 6.75) -> (10.9091, 6.75)
  line L523 (10.9091, 6.75) -> (10.9091, 7.25)
  line L524 (9, 9.25) -> (11.5455, 9.25)
  line L525 (11.5455, 9.25) -> (11.5455, 8.75)
  line L526 (11.5455, 8.75) -> (9, 8.75)
  line L527 (9, 8.75) -> (9, 9.25)
  line L528 (9, 8) -> (16, 8) construction
  line L529 (16, 8) -> (9, 8) construction
  line L530 (13.4545, 5.25) -> (16, 5.25)
  line L531 (16, 5.25) -> (16, 4.75)
  line L532 (16, 4.75) -> (13.4545, 4.75)
  line L533 (13.4545, 4.75) -> (13.4545, 5.25)
  line L534 (10.9091, 3.25) -> (14.0909, 3.25)
  line L535 (14.0909, 3.25) -> (14.0909, 2.75)
  line L536 (14.0909, 2.75) -> (10.9091, 2.75)
  line L537 (10.9091, 2.75) -> (10.9091, 3.25)
  line L538 (9, 5.25) -> (11.5455, 5.25)
  line L539 (11.5455, 5.25) -> (11.5455, 4.75)
  line L540 (11.5455, 4.75) -> (9, 4.75)
  line L541 (9, 4.75) -> (9, 5.25)
  line L542 (9, 4) -> (16, 4) construction
  line L543 (16, 4) -> (9, 4) construction
  line L544 (13.4545, 1.25) -> (16, 1.25)
  line L545 (16, 1.25) -> (16, 0.75)
  line L546 (16, 0.75) -> (13.4545, 0.75)
  line L547 (13.4545, 0.75) -> (13.4545, 1.25)
  line L548 (10.9091, -0.75) -> (14.0909, -0.75)
  line L549 (14.0909, -0.75) -> (14.0909, -1.25)
  line L550 (14.0909, -1.25) -> (10.9091, -1.25)
  line L551 (10.9091, -1.25) -> (10.9091, -0.75)
  line L552 (9, 1.25) -> (11.5455, 1.25)
  line L553 (11.5455, 1.25) -> (11.5455, 0.75)
  line L554 (11.5455, 0.75) -> (9, 0.75)
  line L555 (9, 0.75) -> (9, 1.25)
  line L556 (9, 0) -> (16, 0) construction
  line L557 (16, 0) -> (9, 0) construction
  line L558 (0.7, 11) -> (7.7, 11)
  line L559 (7.7, 11) -> (7.7, -11)
  line L560 (7.7, -11) -> (0.7, -11)
  line L561 (0.7, -11) -> (0.7, 11)
  line L562 (0.7, 1.25) -> (3.2455, 1.25)
  line L563 (3.2455, 1.25) -> (3.2455, 0.75)
  line L564 (3.2455, 0.75) -> (0.7, 0.75)
  line L565 (0.7, 0.75) -> (0.7, 1.25)
  line L566 (5.1545, 0.75) -> (5.1545, 1.25)
  line L567 (7.7, 0.75) -> (5.1545, 0.75)
  line L568 (5.1545, 1.25) -> (7.7, 1.25)
  line L569 (7.7, 1.25) -> (7.7, 0.75)
  line L570 (2.6091, -0.75) -> (5.7909, -0.75)
  line L571 (5.7909, -0.75) -> (5.7909, -1.25)
  line L572 (5.7909, -1.25) -> (2.6091, -1.25)
  line L573 (2.6091, -1.25) -> (2.6091, -0.75)
  line L574 (0.7, 0) -> (7.7, 0) construction
  line L575 (7.7, 0) -> (0.7, 0) construction
  line L576 (5.1545, -2.75) -> (7.7, -2.75)
  line L577 (7.7, -2.75) -> (7.7, -3.25)
  line L578 (7.7, -3.25) -> (5.1545, -3.25)
  line L579 (5.1545, -3.25) -> (5.1545, -2.75)
  line L580 (2.6091, -4.75) -> (5.7909, -4.75)
  line L581 (5.7909, -4.75) -> (5.7909, -5.25)
  line L582 (5.7909, -5.25) -> (2.6091, -5.25)
  line L583 (2.6091, -5.25) -> (2.6091, -4.75)
  line L584 (0.7, -2.75) -> (3.2455, -2.75)
  line L585 (3.2455, -2.75) -> (3.2455, -3.25)
  line L586 (3.2455, -3.25) -> (0.7, -3.25)
  line L587 (0.7, -3.25) -> (0.7, -2.75)
  line L588 (0.7, -4) -> (7.7, -4) construction
  line L589 (7.7, -4) -> (0.7, -4) construction
  line L590 (5.1545, -6.75) -> (7.7, -6.75)
  line L591 (7.7, -6.75) -> (7.7, -7.25)
  line L592 (7.7, -7.25) -> (5.1545, -7.25)
  line L593 (5.1545, -7.25) -> (5.1545, -6.75)
  line L594 (2.6091, -8.75) -> (5.7909, -8.75)
  line L595 (5.7909, -8.75) -> (5.7909, -9.25)
  line L596 (5.7909, -9.25) -> (2.6091, -9.25)
  line L597 (2.6091, -9.25) -> (2.6091, -8.75)
  line L598 (0.7, -6.75) -> (3.2455, -6.75)
  line L599 (3.2455, -6.75) -> (3.2455, -7.25)
  line L600 (3.2455, -7.25) -> (0.7, -7.25)
  line L601 (0.7, -7.25) -> (0.7, -6.75)
  line L602 (0.7, -8) -> (7.7, -8) construction
  line L603 (7.7, -8) -> (0.7, -8) construction
  line L604 (5.1545, 5.25) -> (7.7, 5.25)
  line L605 (7.7, 5.25) -> (7.7, 4.75)
  line L606 (7.7, 4.75) -> (5.1545, 4.75)
  line L607 (5.1545, 4.75) -> (5.1545, 5.25)
  line L608 (2.6091, 3.25) -> (5.7909, 3.25)
  line L609 (5.7909, 3.25) -> (5.7909, 2.75)
  line L610 (5.7909, 2.75) -> (2.6091, 2.75)
  line L611 (2.6091, 2.75) -> (2.6091, 3.25)
  line L612 (0.7, 5.25) -> (3.2455, 5.25)
  line L613 (3.2455, 5.25) -> (3.2455, 4.75)
  line L614 (3.2455, 4.75) -> (0.7, 4.75)
  line L615 (0.7, 4.75) -> (0.7, 5.25)
  line L616 (0.7, 4) -> (7.7, 4) construction
  line L617 (7.7, 4) -> (0.7, 4) construction
  line L618 (5.1545, 1.25) -> (7.7, 1.25)
  line L619 (7.7, 1.25) -> (7.7, 0.75)
  line L620 (7.7, 0.75) -> (5.1545, 0.75)
  line L621 (5.1545, 0.75) -> (5.1545, 1.25)
  line L622 (2.6091, -0.75) -> (5.7909, -0.75)
  line L623 (5.7909, -0.75) -> (5.7909, -1.25)
  line L624 (5.7909, -1.25) -> (2.6091, -1.25)
  line L625 (2.6091, -1.25) -> (2.6091, -0.75)
  line L626 (0.7, 1.25) -> (3.2455, 1.25)
  line L627 (3.2455, 1.25) -> (3.2455, 0.75)
  line L628 (3.2455, 0.75) -> (0.7, 0.75)
  line L629 (0.7, 0.75) -> (0.7, 1.25)
  line L630 (0.7, 0) -> (7.7, 0) construction
  line L631 (7.7, 0) -> (0.7, 0) construction
  line L632 (5.1545, -2.75) -> (7.7, -2.75)
  line L633 (7.7, -2.75) -> (7.7, -3.25)
  line L634 (7.7, -3.25) -> (5.1545, -3.25)
  line L635 (5.1545, -3.25) -> (5.1545, -2.75)
  line L636 (2.6091, -4.75) -> (5.7909, -4.75)
  line L637 (5.7909, -4.75) -> (5.7909, -5.25)
  line L638 (5.7909, -5.25) -> (2.6091, -5.25)
  line L639 (2.6091, -5.25) -> (2.6091, -4.75)
  line L640 (0.7, -2.75) -> (3.2455, -2.75)
  line L641 (3.2455, -2.75) -> (3.2455, -3.25)
  line L642 (3.2455, -3.25) -> (0.7, -3.25)
  line L643 (0.7, -3.25) -> (0.7, -2.75)
  line L644 (0.7, -4) -> (7.7, -4) construction
  line L645 (7.7, -4) -> (0.7, -4) construction
  line L646 (5.1545, 9.25) -> (7.7, 9.25)
  line L647 (7.7, 9.25) -> (7.7, 8.75)
  line L648 (7.7, 8.75) -> (5.1545, 8.75)
  line L649 (5.1545, 8.75) -> (5.1545, 9.25)
  line L650 (2.6091, 7.25) -> (5.7909, 7.25)
  line L651 (5.7909, 7.25) -> (5.7909, 6.75)
  line L652 (5.7909, 6.75) -> (2.6091, 6.75)
  line L653 (2.6091, 6.75) -> (2.6091, 7.25)
  line L654 (0.7, 9.25) -> (3.2455, 9.25)
  line L655 (3.2455, 9.25) -> (3.2455, 8.75)
  line L656 (3.2455, 8.75) -> (0.7, 8.75)
  line L657 (0.7, 8.75) -> (0.7, 9.25)
  line L658 (0.7, 8) -> (7.7, 8) construction
  line L659 (7.7, 8) -> (0.7, 8) construction
  line L660 (5.1545, 5.25) -> (7.7, 5.25)
  line L661 (7.7, 5.25) -> (7.7, 4.75)
  line L662 (7.7, 4.75) -> (5.1545, 4.75)
  line L663 (5.1545, 4.75) -> (5.1545, 5.25)
  line L664 (2.6091, 3.25) -> (5.7909, 3.25)
  line L665 (5.7909, 3.25) -> (5.7909, 2.75)
  line L666 (5.7909, 2.75) -> (2.6091, 2.75)
  line L667 (2.6091, 2.75) -> (2.6091, 3.25)
  line L668 (0.7, 5.25) -> (3.2455, 5.25)
  line L669 (3.2455, 5.25) -> (3.2455, 4.75)
  line L670 (3.2455, 4.75) -> (0.7, 4.75)
  line L671 (0.7, 4.75) -> (0.7, 5.25)
  line L672 (0.7, 4) -> (7.7, 4) construction
  line L673 (7.7, 4) -> (0.7, 4) construction
  line L674 (5.1545, 1.25) -> (7.7, 1.25)
  line L675 (7.7, 1.25) -> (7.7, 0.75)
  line L676 (7.7, 0.75) -> (5.1545, 0.75)
  line L677 (5.1545, 0.75) -> (5.1545, 1.25)
  line L678 (2.6091, -0.75) -> (5.7909, -0.75)
  line L679 (5.7909, -0.75) -> (5.7909, -1.25)
  line L680 (5.7909, -1.25) -> (2.6091, -1.25)
  line L681 (2.6091, -1.25) -> (2.6091, -0.75)
  line L682 (0.7, 1.25) -> (3.2455, 1.25)
  line L683 (3.2455, 1.25) -> (3.2455, 0.75)
  line L684 (3.2455, 0.75) -> (0.7, 0.75)
  line L685 (0.7, 0.75) -> (0.7, 1.25)
  line L686 (0.7, 0) -> (7.7, 0) construction
  line L687 (7.7, 0) -> (0.7, 0) construction
  line L688 (5.1545, -10.75) -> (7.7, -10.75)
  line L689 (7.7, -10.75) -> (7.7, -11.25)
  line L690 (7.7, -11.25) -> (5.1545, -11.25)
  line L691 (5.1545, -11.25) -> (5.1545, -10.75)
  line L692 (2.6091, -12.75) -> (5.7909, -12.75)
  line L693 (5.7909, -12.75) -> (5.7909, -13.25)
  line L694 (5.7909, -13.25) -> (2.6091, -13.25)
  line L695 (2.6091, -13.25) -> (2.6091, -12.75)
  line L696 (0.7, -10.75) -> (3.2455, -10.75)
  line L697 (3.2455, -10.75) -> (3.2455, -11.25)
  line L698 (3.2455, -11.25) -> (0.7, -11.25)
  line L699 (0.7, -11.25) -> (0.7, -10.75)
  line L700 (0.7, -12) -> (7.7, -12) construction
  line L701 (7.7, -12) -> (0.7, -12) construction
  line L702 (5.1545, -6.75) -> (7.7, -6.75)
  line L703 (7.7, -6.75) -> (7.7, -7.25)
  line L704 (7.7, -7.25) -> (5.1545, -7.25)
  line L705 (5.1545, -7.25) -> (5.1545, -6.75)
  line L706 (2.6091, -8.75) -> (5.7909, -8.75)
  line L707 (5.7909, -8.75) -> (5.7909, -9.25)
  line L708 (5.7909, -9.25) -> (2.6091, -9.25)
  line L709 (2.6091, -9.25) -> (2.6091, -8.75)
  line L710 (0.7, -6.75) -> (3.2455, -6.75)
  line L711 (3.2455, -6.75) -> (3.2455, -7.25)
  line L712 (3.2455, -7.25) -> (0.7, -7.25)
  line L713 (0.7, -7.25) -> (0.7, -6.75)
  line L714 (0.7, -8) -> (7.7, -8) construction
  line L715 (7.7, -8) -> (0.7, -8) construction
  line L716 (5.1545, -2.75) -> (7.7, -2.75)
  line L717 (7.7, -2.75) -> (7.7, -3.25)
  line L718 (7.7, -3.25) -> (5.1545, -3.25)
  line L719 (5.1545, -3.25) -> (5.1545, -2.75)
  line L720 (2.6091, -4.75) -> (5.7909, -4.75)
  line L721 (5.7909, -4.75) -> (5.7909, -5.25)
  line L722 (5.7909, -5.25) -> (2.6091, -5.25)
  line L723 (2.6091, -5.25) -> (2.6091, -4.75)
  line L724 (0.7, -2.75) -> (3.2455, -2.75)
  line L725 (3.2455, -2.75) -> (3.2455, -3.25)
  line L726 (3.2455, -3.25) -> (0.7, -3.25)
  line L727 (0.7, -3.25) -> (0.7, -2.75)
  line L728 (0.7, -4) -> (7.7, -4) construction
  line L729 (7.7, -4) -> (0.7, -4) construction
  line L730 (5.1545, 13.25) -> (7.7, 13.25)
  line L731 (7.7, 13.25) -> (7.7, 12.75)
  line L732 (7.7, 12.75) -> (5.1545, 12.75)
  line L733 (5.1545, 12.75) -> (5.1545, 13.25)
  line L734 (2.6091, 11.25) -> (5.7909, 11.25)
  line L735 (5.7909, 11.25) -> (5.7909, 10.75)
  line L736 (5.7909, 10.75) -> (2.6091, 10.75)
  line L737 (2.6091, 10.75) -> (2.6091, 11.25)
  line L738 (0.7, 13.25) -> (3.2455, 13.25)
  line L739 (3.2455, 13.25) -> (3.2455, 12.75)
  line L740 (3.2455, 12.75) -> (0.7, 12.75)
  line L741 (0.7, 12.75) -> (0.7, 13.25)
  line L742 (0.7, 12) -> (7.7, 12) construction
  line L743 (7.7, 12) -> (0.7, 12) construction
  line L744 (5.1545, 9.25) -> (7.7, 9.25)
  line L745 (7.7, 9.25) -> (7.7, 8.75)
  line L746 (7.7, 8.75) -> (5.1545, 8.75)
  line L747 (5.1545, 8.75) -> (5.1545, 9.25)
  line L748 (2.6091, 7.25) -> (5.7909, 7.25)
  line L749 (5.7909, 7.25) -> (5.7909, 6.75)
  line L750 (5.7909, 6.75) -> (2.6091, 6.75)
  line L751 (2.6091, 6.75) -> (2.6091, 7.25)
  line L752 (0.7, 9.25) -> (3.2455, 9.25)
  line L753 (3.2455, 9.25) -> (3.2455, 8.75)
  line L754 (3.2455, 8.75) -> (0.7, 8.75)
  line L755 (0.7, 8.75) -> (0.7, 9.25)
  line L756 (0.7, 8) -> (7.7, 8) construction
  line L757 (7.7, 8) -> (0.7, 8) construction
  line L758 (5.1545, 5.25) -> (7.7, 5.25)
  line L759 (7.7, 5.25) -> (7.7, 4.75)
  line L760 (7.7, 4.75) -> (5.1545, 4.75)
  line L761 (5.1545, 4.75) -> (5.1545, 5.25)
  line L762 (2.6091, 3.25) -> (5.7909, 3.25)
  line L763 (5.7909, 3.25) -> (5.7909, 2.75)
  line L764 (5.7909, 2.75) -> (2.6091, 2.75)
  line L765 (2.6091, 2.75) -> (2.6091, 3.25)
  line L766 (0.7, 5.25) -> (3.2455, 5.25)
  line L767 (3.2455, 5.25) -> (3.2455, 4.75)
  line L768 (3.2455, 4.75) -> (0.7, 4.75)
  line L769 (0.7, 4.75) -> (0.7, 5.25)
  line L770 (0.7, 4) -> (7.7, 4) construction
  line L771 (7.7, 4) -> (0.7, 4) construction
  line L772 (5.1545, 1.25) -> (7.7, 1.25)
  line L773 (7.7, 1.25) -> (7.7, 0.75)
  line L774 (7.7, 0.75) -> (5.1545, 0.75)
  line L775 (5.1545, 0.75) -> (5.1545, 1.25)
  line L776 (2.6091, -0.75) -> (5.7909, -0.75)
  line L777 (5.7909, -0.75) -> (5.7909, -1.25)